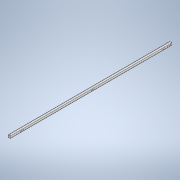
# Autodesk Inventor part: プレート保持_角柱1
Saved by Autodesk Inventor 2021 (Build 250183000, 183)
## iProperties
Created: 2022-02-03
Part Number: プレート保持_角柱1
Material: 一般
Document SubType Name: Modeling
Designer: hirohumi
Density: 1 g/cm^3
Appearance: 既定
Author: hirohumi
Autodesk Inventor part; units mm, degrees
ref_plane "YZ Plane" through (0, 0, 0) normal (1, 0, 0) x (0, 1, 0)
ref_plane "XZ Plane" through (0, 0, 0) normal (0, 1, 0) x (-1, 0, 0)
ref_plane "XY Plane" through (0, 0, 0) normal (0, 0, 1) x (1, 0, 0)
sketch "スケッチ1" plane through (0, 0, 0) normal (0, 0, 1) x (1, 0, 0)
  line L0 (7.5, 7.5) -> (-7.5, 7.5)
  line L1 (-7.5, 7.5) -> (-7.5, -7.5)
  line L2 (-7.5, -7.5) -> (7.5, -7.5)
  line L3 (7.5, -7.5) -> (7.5, 7.5)
  line L4 (7.5, 7.5) -> (-7.5, -7.5) construction
  line L5 (-7.5, 7.5) -> (7.5, -7.5) construction
  line L6 (-6.5, 6.5) -> (6.5, 6.5)
  line L7 (6.5, 6.5) -> (6.5, -6.5)
  line L8 (6.5, -6.5) -> (-6.5, -6.5)
  line L9 (-6.5, -6.5) -> (-6.5, 6.5)
  point P0 (0, 0)
  dimension "d0" = 15
  dimension "d1" = 15
  dimension "d2" = 1
  constraints: 20 end point, 4 parallel, 2 midpoint, 2 perpendicular, 1 horizontal, 3 other
  measures "d0" distance of L2.end L1.end
  measures "d1" distance of L1.end L0.end
  measures "d2" distance between parallel lines of L0 L6
extrude "押し出し1" add sketch "スケッチ1" along normal blind 1142
sketch "スケッチ2" plane through (7.5, 7.5, 1142) normal (1, 0, 0) x (0, 0, -1)
  circle A0 centre (1132, -7.5) radius 1.6
  circle A1 centre (1122, -7.5) radius 1.6
  circle A2 centre (1112, -7.5) radius 1.6
  line L0 (1142, -15) -> (1142, 0) projected
  circle A3 centre (592, -7.5) radius 1.6
  circle A4 centre (582, -7.5) radius 1.6
  circle A5 centre (572, -7.5) radius 1.6
  circle A6 centre (1092, -7.5) radius 1.6
  circle A7 centre (1082, -7.5) radius 1.6
  circle A8 centre (1072, -7.5) radius 1.6
  circle A9 centre (92, -7.5) radius 1.6
  circle A10 centre (82, -7.5) radius 1.6
  circle A11 centre (72, -7.5) radius 1.6
  point P0 (1142, -7.5)
  point P1 (1142, -7.5)
  dimension "d5" = 3.2
  dimension "d6" = 3.2
  dimension "d7" = 3.2
  dimension "d8" = 10
  dimension "d9" = 10
  dimension "d10" = 10
  dimension "d11" = 3.2
  dimension "d12" = 3.2
  dimension "d13" = 3.2
  dimension "d14" = 10
  dimension "d15" = 10
  dimension "d25" = 3.2
  dimension "d26" = 3.2
  dimension "d27" = 3.2
  dimension "d28" = 10
  dimension "d29" = 10
  dimension "d30" = 20
  dimension "d31" = 500
  dimension "d32" = 3.2
  dimension "d33" = 3.2
  dimension "d34" = 3.2
  dimension "d35" = 10
  dimension "d36" = 10
  dimension "d37" = 500
  constraints: 12 centre point, 12 horizontal alignment, 1 midpoint
  measures "d5" diameter of A0
  measures "d6" diameter of A1
  measures "d7" diameter of A2
  measures "d8" distance of point (1142, -7.5) A0.centre
  measures "d9" distance of A0.centre A1.centre
  measures "d10" distance of A1.centre A2.centre
  measures "d11" diameter of A3
  measures "d12" diameter of A4
  measures "d13" diameter of A5
  measures "d14" distance of A3.centre A4.centre
  measures "d15" distance of A4.centre A5.centre
  measures "d25" diameter of A6
  measures "d26" diameter of A7
  measures "d27" diameter of A8
  measures "d28" distance of A7.centre A8.centre
  measures "d29" distance of A6.centre A7.centre
  measures "d30" distance of A2.centre A6.centre
  measures "d31" distance of A7.centre A4.centre
  measures "d32" diameter of A9
  measures "d33" diameter of A10
  measures "d34" diameter of A11
  measures "d35" distance of A9.centre A10.centre
  measures "d36" distance of A10.centre A11.centre
  measures "d37" distance of A4.centre A10.centre
extrude "押し出し2" cut sketch "スケッチ2" against normal through all
sketch "スケッチ3" plane through (-7.5, 7.5, 1142) normal (0, 1, 0) x (1, 0, 0)
  circle A0 centre (7.5, 7.5) radius 1.6
  line L0 (0, 1142) -> (0, 0) projected
  line L1 (15, 0) -> (0, 0) projected
  point P0 (7.5, 1142)
  dimension "d19" = 3.2
  dimension "d20" = 7.5
  dimension "d21" = 7.5
  constraints: 1 centre point
  measures "d19" diameter of A0
  measures "d20" distance from line of L0 A0.centre
  measures "d21" distance from line of L1 A0.centre
extrude "押し出し3" cut sketch "スケッチ3" against normal through all
